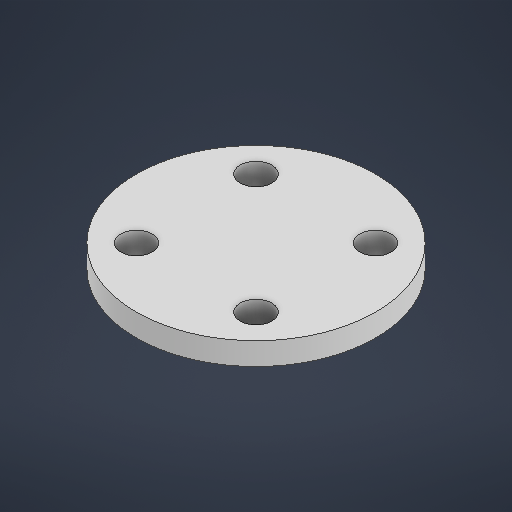
# Autodesk Inventor part: WristSpaacer
Saved by Autodesk Inventor 2025 (Build 290162000, 162)
## iProperties
Created: 2024-05-22
Part Number: WristSpaacer
Material: Generic
Document SubType Name: Modeling
Designer: avsar
Density: 1 g/cm^3
Appearance: Default
Author: avsar
Autodesk Inventor part; units mm, degrees
ref_plane "YZ Plane" through (0, 0, 0) normal (1, 0, 0) x (0, 1, 0)
ref_plane "XZ Plane" through (0, 0, 0) normal (0, 1, 0) x (-1, 0, 0)
ref_plane "XY Plane" through (0, 0, 0) normal (0, 0, 1) x (1, 0, 0)
sketch "Sketch1" plane through (0, 0, 0) normal (0, 1, 0) x (-1, 0, 0)
  circle A0 centre (0, 0) radius 16
  circle A1 centre (8, -8) radius 2.1
  circle A2 centre (8, 8) radius 2.1
  circle A3 centre (-8, 8) radius 2.1
  circle A4 centre (-8, -8) radius 2.1
  dimension "d0" = 32
  dimension "d1" = 4.2
  dimension "d2" = 8
  dimension "d3" = 8
  dimension "d6" = 360
  constraints: 5 centre point, 1 coincident, 9 other
  measures "d0" diameter of A0
  measures "d1" diameter of A1
  measures "d2" horizontal distance of point (0, 0) A1.centre
  measures "d3" horizontal distance of point (0, 0) A1.centre
extrude "Extrusion1" add sketch "Sketch1" along normal blind 3
body "Solid1"
